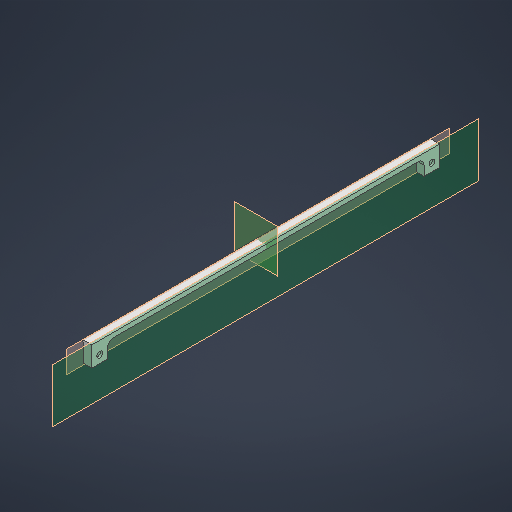
# Autodesk Inventor part: Spcer_Upper
Saved by Autodesk Inventor 2026.3 (Build 303398000, 398)
## iProperties
Created: 2026-09-07
Part Number: Spcer_Upper
Material: 一般
Document SubType Name: Modeling
Designer: takuya
Density: 1 g/cm^3
Appearance: 既定
Author: takuya
Autodesk Inventor part; units mm, degrees
ref_plane "YZ Plane" through (0, 0, 0) normal (1, 0, 0) x (0, 1, 0)
ref_plane "XZ Plane" through (0, 0, 0) normal (0, 1, 0) x (-1, 0, 0)
sketch "スケッチ1" plane through (0, 0, 0) normal (0, 0, 1) x (1, 0, 0)
  line L0 (-53.8577, -21) -> (53.8577, -21) projected
  line L1 (53.8577, -21) -> (53.8577, 21) projected
  line L2 (53.8577, 21) -> (48.8577, 21) projected
  line L3 (48.8577, 21) -> (49.7747, 18.6743) projected
  line L4 (49.7747, 18.6743) -> (-44.506, -18.5) projected
  line L5 (-44.506, -18.5) -> (-45.423, -16.1743) projected
  line L6 (-45.423, -16.1743) -> (-53.8577, -19.5) projected
  line L7 (-53.8577, -19.5) -> (-53.8577, -21) projected
  line L8 (-14.7433, -12.1394) -> (42.0411, 10.2503) projected
  arc A0 (44.7747, 8.3897) -> (42.0411, 10.2503) centre (42.7747, 8.3897) ccw projected
  line L9 (44.7747, 8.3897) -> (44.7747, -14) projected
  arc A1 (42.7747, -16) -> (44.7747, -14) centre (42.7747, -14) ccw projected
  line L10 (42.7747, -16) -> (-14.0097, -16) projected
  arc A2 (-14.7433, -12.1394) -> (-14.0097, -16) centre (-14.0097, -14) ccw projected
  line L11 (49.7747, 18.6743) -> (53.8577, 18.6743)
  point P0 (0, 0)
  constraints: 2 end point, 1 perpendicular, 1 point on line
ref_plane "作業平面1" through (-53.8577, -21, 178) normal (0, 0, -1) x (0, 1, 0)
extrude "押し出し1" add sketch "スケッチ1" along normal up to surface (178 mm away) contours L11 L3 L2 L1
ref_plane "作業平面2" through (53.8577, 21, -10) normal (-1, 0, 0) x (0, 1, 0)
sketch "スケッチ3" plane through (53.8577, 21, -10) normal (-1, 0, 0) x (0, 1, 0)
  line L0 (-2.3257, -10) -> (-2.3257, -188) projected
  line L1 (-2.3257, -10) -> (0, -10) projected
  line L2 (-2.3257, -10) -> (-10.3257, -10)
  line L3 (-10.3257, -10) -> (-10.3257, -18)
  line L4 (-10.3257, -18) -> (-2.3257, -18)
  line L5 (-2.3257, -18) -> (-2.3257, -10)
  circle A0 centre (-6.3257, -14) radius 1.5
  line L6 (-3.4757, -15.6454) -> (-6.3257, -17.2909)
  line L7 (-6.3257, -17.2909) -> (-9.1757, -15.6454)
  line L8 (-9.1757, -15.6454) -> (-9.1757, -12.3546)
  line L9 (-9.1757, -12.3546) -> (-6.3257, -10.7091)
  line L10 (-6.3257, -10.7091) -> (-3.4757, -12.3546)
  line L11 (-3.4757, -12.3546) -> (-3.4757, -15.6454)
  point P0 (-21, -10)
  dimension "d5" = 8
  dimension "d6" = 8
  dimension "d7" = 3
  dimension "d8" = 5.7
  constraints: 20 end point, 2 parallel, 1 centre point, 1 coincident, 1 horizontal, 1 perpendicular, 13 other
  measures "d5" distance of L4.end L3.end
  measures "d6" distance of L3.end L2.end
  measures "d7" diameter of A0
  measures "d8" distance between parallel lines of L8 L11
extrude "押し出し2" add sketch "スケッチ3" along normal blind 4.083 contours L0 L4 L3 L2 | L6 L7 L8 L9 L10 L11
ref_plane "作業平面4" through (49.7747, 18.6743, 0) normal (1, 0, 0) x (0, 0, -1)
sketch "スケッチ4" plane through (49.7747, 21, -10) normal (-1, 0, 0) x (0, 0, 1)
  circle A0 centre (14, -6.3257) radius 1.5 projected
  line L0 (12.3546, -9.1757) -> (10.7091, -6.3257)
  line L1 (10.7091, -6.3257) -> (12.3546, -3.4757)
  line L2 (12.3546, -3.4757) -> (15.6454, -3.4757)
  line L3 (15.6454, -3.4757) -> (17.2909, -6.3257)
  line L4 (17.2909, -6.3257) -> (15.6454, -9.1757)
  line L5 (15.6454, -9.1757) -> (12.3546, -9.1757)
  point P0 (10, -21)
  point P1 (14, -3.4757)
  point P2 (14, -9.1757)
  dimension "d11" = 5.7
  constraints: 12 end point, 2 midpoint, 1 coincident, 13 other
  measures "d11" distance of point (14, -3.476) point (14, -9.176)
extrude "押し出し3" cut sketch "スケッチ4" against normal blind 3
sketch "スケッチ5" plane through (49.7747, 21, -10) normal (-1, 0, 0) x (0, 0, 1)
  line L0 (18, -2.3257) -> (10, -2.3257) projected
  line L1 (18, -2.3257) -> (188, -2.3257) projected
  line L2 (18, -10.3257) -> (18, -2.3257) projected
  line L3 (18, -2.3257) -> (21, -2.3257)
  line L4 (21, -2.3257) -> (21, -5.3257)
  line L5 (21, -5.3257) -> (18, -5.3257)
  line L6 (18, -5.3257) -> (18, -2.3257)
  arc A0 (21, -2.3257) -> (18, -5.3257) centre (21, -5.3257) ccw
  point P0 (10, -21)
  point P1 (21, -2.3257)
  dimension "d14" = 3
  dimension "d15" = 3
  constraints: 8 end point, 2 parallel, 2 point on circle, 1 centre point, 1 horizontal, 1 perpendicular, 1 tangent
  measures "d14" distance of L3.end L4.end
  measures "d15" distance of L4.end L5.end
extrude "押し出し4" add sketch "スケッチ5" against normal blind 4.083 contours L1 A0 L2
ref_plane "作業平面5" through (48.8577, 21, 89) normal (0, 0, 1) x (1, 0, 0)
mirror "ミラー1" about plane through (48.8577, 21, 89) normal (0, 0, 1) of "押し出し2", "押し出し4"
mirror "ミラー2" about plane through (48.8577, 21, 89) normal (0, 0, 1) of "押し出し3"
ref_plane "作業平面6" through (48.8577, 21, 89) normal (0, 0, 1) x (1, 0, 0)
equation "\"d6\" = d5"
